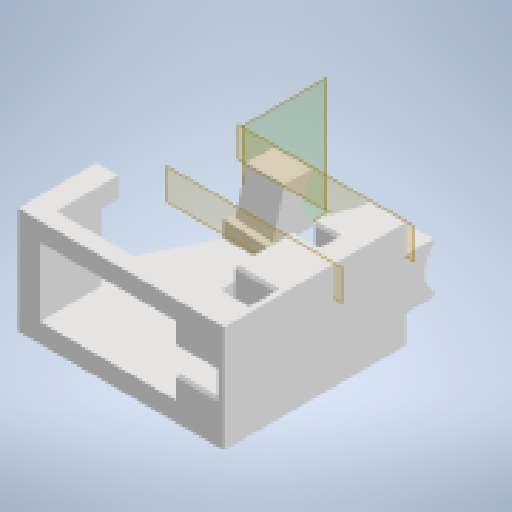
# Autodesk Inventor part: Servo Mount
Saved by Autodesk Inventor 2024 (Build 280153000, 153)
## iProperties
Created: 2024-11-25
Part Number: Servo Mount
Material: Generic
Document SubType Name: Modeling
Designer: Tommy Rohmann
Density: 1 g/cm^3
Appearance: Default
Author: Tommy Rohmann
Autodesk Inventor part; units mm, degrees
sketch "Servo Footprint" plane through (0, 0, 0) normal (0, 0, 1) x (1, 0, 0)
  line L0 (-70.3478, -47.479) -> (-30.4698, -47.479)
  line L1 (-30.4698, -47.479) -> (-30.4698, -27.667)
  line L2 (-30.4698, -27.667) -> (-70.3478, -27.667)
  line L3 (-70.3478, -47.479) -> (-30.4698, -27.667) construction
  line L4 (-30.4698, -47.479) -> (-70.3478, -27.667) construction
  line L5 (-77.5868, -47.479) -> (-23.2308, -47.479)
  line L6 (-23.2308, -47.479) -> (-23.2308, -27.667)
  line L7 (-23.2308, -27.667) -> (-77.5868, -27.667)
  line L8 (-77.5868, -47.479) -> (-23.2308, -27.667) construction
  line L9 (-23.2308, -47.479) -> (-77.5868, -27.667) construction
  line L10 (-30.4698, -37.573) -> (-39.8678, -37.573)
  line L11 (-77.5868, -47.479) -> (-77.5868, -27.667)
  line L12 (-70.3478, -27.667) -> (-70.3478, -47.479)
  point P0 (-45.544, -37.573)
  point P1 (-50.4088, -37.573)
  point P2 (-50.4088, -37.573)
  dimension "d0" = 39.878
  dimension "d1" = 19.812
  dimension "d2" = 54.356
  dimension "d3" = 9.398
  measures "d0" distance of L0.start L0.end
  measures "d1" distance of L1.end L0.end
  measures "d2" distance of L5.start L5.end
  measures "d3" distance of L10.start L10.end
sketch "Valve Casing" plane through (0, 0, 0) normal (0, 0, 1) x (1, 0, 0)
  circle A0 centre (0, 0) radius 8.636
  circle A1 centre (0, 0) radius 11.176
  circle A2 centre (0, 0) radius 12.446
  dimension "d30" = 24.892
  measures "d30" diameter of A2
sketch "Servo Arm Socket" plane through (0, 0, 0) normal (0, 0, 1) x (1, 0, 0)
  arc A0 (4.8166, -0.3016) -> (-4.8166, -0.3016) centre (0, 0) ccw
  line L0 (0, 0) -> (0, -20.32)
  arc A1 (-3.549, -20.5423) -> (3.549, -20.5423) centre (0, -20.32) ccw
  line L1 (-3.549, -20.5423) -> (-4.8166, -0.3016)
  line L2 (4.8166, -0.3016) -> (3.549, -20.5423)
  line L3 (-5.0701, -0.3175) -> (-3.8026, -20.5581)
  arc A2 (-3.8026, -20.5581) -> (3.8026, -20.5581) centre (0, -20.32) ccw
  line L4 (3.8026, -20.5581) -> (5.0701, -0.3175)
  arc A3 (5.0701, -0.3175) -> (-5.0701, -0.3175) centre (0, 0) ccw
  line L5 (-6.3376, -20.7169) -> (-7.6051, -0.4762)
  arc A4 (7.6051, -0.4763) -> (-7.6051, -0.4762) centre (0, 0) ccw
  line L6 (7.6051, -0.4763) -> (6.3376, -20.7169)
  arc A5 (-6.3376, -20.7169) -> (6.3376, -20.7169) centre (0, -20.32) ccw
  dimension "d0" = 39.878
  dimension "d1" = 19.812
  dimension "d2" = 54.356
  dimension "d3" = 9.398
  dimension "d39" = 9.652
  dimension "d40" = 20.32
  dimension "d41" = 7.112
  dimension "d42" = 0.254
  dimension "d43" = 2.54
  measures "d39" diameter of A0
  measures "d40" distance of L0.start L0.end
  measures "d41" diameter of A1
  measures "d42" distance between parallel lines of L1 L3
  measures "d43" distance between parallel lines of L3 L5
sketch "Most Annoying thing Possibly Ever" plane through (0, 0, 0) normal (0, 0, 1) x (1, 0, 0)
  line L0 (1.9811, 57.7148) -> (1.9811, 71.8118)
  line L1 (16.0781, 71.8118) -> (1.9811, 71.8118)
  arc A0 (1.9811, 45.1418) -> (28.6511, 71.8118) centre (1.9811, 71.8118) ccw
  arc A1 (1.9811, 44.6338) -> (29.1591, 71.8118) centre (1.9811, 71.8118) ccw
  circle A2 centre (1.9811, 71.8118) radius 8.636
  circle A3 centre (1.9811, 71.8118) radius 11.176
  circle A4 centre (1.9811, 71.8118) radius 12.446
  arc A5 (6.7977, 71.5101) -> (-2.8354, 71.5101) centre (1.9811, 71.8118) ccw
  line L2 (1.9811, 71.8118) -> (1.9811, 51.4918)
  arc A6 (-1.5679, 51.2695) -> (5.5302, 51.2695) centre (1.9811, 51.4918) ccw
  line L3 (-1.5679, 51.2695) -> (-2.8354, 71.5101)
  line L4 (6.7977, 71.5101) -> (5.5302, 51.2695)
  line L5 (-3.0889, 71.4943) -> (-1.8214, 51.2536)
  arc A7 (-1.8214, 51.2536) -> (5.7837, 51.2536) centre (1.9811, 51.4918) ccw
  line L6 (5.7837, 51.2536) -> (7.0512, 71.4943)
  arc A8 (7.0512, 71.4943) -> (-3.0889, 71.4943) centre (1.9811, 71.8118) ccw
  line L7 (-4.3564, 51.0949) -> (-5.624, 71.3355)
  arc A9 (9.5862, 71.3355) -> (-5.624, 71.3355) centre (1.9811, 71.8118) ccw
  line L8 (9.5862, 71.3355) -> (8.3187, 51.0949)
  arc A10 (-4.3564, 51.0949) -> (8.3187, 51.0949) centre (1.9811, 51.4918) ccw
  arc A11 (2.2828, 76.6283) -> (2.2828, 66.9952) centre (1.9811, 71.8118) ccw
  line L9 (1.9811, 71.8118) -> (22.3011, 71.8118)
  arc A12 (22.5234, 68.2627) -> (22.5234, 75.3608) centre (22.3011, 71.8118) ccw
  line L10 (22.5234, 68.2627) -> (2.2828, 66.9952)
  line L11 (2.2828, 76.6283) -> (22.5234, 75.3608)
  line L12 (2.2986, 66.7417) -> (22.5393, 68.0092)
  arc A13 (22.5393, 68.0092) -> (22.5393, 75.6143) centre (22.3011, 71.8118) ccw
  line L13 (22.5393, 75.6143) -> (2.2986, 76.8818)
  arc A14 (2.2986, 76.8818) -> (2.2986, 66.7417) centre (1.9811, 71.8118) ccw
  line L14 (22.698, 65.4742) -> (2.4574, 64.2067)
  arc A15 (2.4574, 79.4169) -> (2.4574, 64.2067) centre (1.9811, 71.8118) ccw
  line L15 (2.4574, 79.4169) -> (22.698, 78.1493)
  arc A16 (22.698, 65.4742) -> (22.698, 78.1493) centre (22.3011, 71.8118) ccw
  point P0 (7.2472, 66.5457)
  point P1 (1.9811, 48.0247)
  point P2 (25.7682, 71.8118)
  dimension "d61" = 0.508
  measures "d61" radial gap between concentric circles of A0 A1
ref_plane "Work Plane1" through (0, 23.3934, 0) normal (0, 0, 1) x (1, 0, 0)
sketch "Sketch1" plane through (0, 23.3934, 0) normal (0, 0, 1) x (1, 0, 0)
  line L0 (-11.8935, 4.1783) -> (-11.8935, -4.1783) projected
  line L1 (-11.8935, -4.1783) -> (1.6581, -4.1783) projected
  arc A0 (22.129, -4.1783) -> (1.6581, -4.1783) centre (11.8935, -11.6967) ccw projected
  line L2 (35.6806, -4.1783) -> (22.129, -4.1783) projected
  line L3 (35.6806, 4.1783) -> (35.6806, -4.1783) projected
  line L4 (-11.8935, 4.1783) -> (35.6806, 4.1783) projected
  arc A1 (1.6581, -19.2151) -> (22.129, -19.2151) centre (11.8935, -11.6967) ccw projected
  line L5 (1.6581, -19.2151) -> (-11.8935, -19.2151) projected
  line L6 (-11.8935, -19.2151) -> (-11.8936, -27.5717) projected
  line L7 (-11.8936, -27.5717) -> (35.6806, -27.5717) projected
  line L8 (35.6806, -19.2151) -> (35.6806, -27.5717) projected
  line L9 (22.129, -19.2151) -> (35.6806, -19.2151) projected
  line L10 (35.6806, -19.2151) -> (35.6806, -4.1783) projected
  line L11 (-11.8935, -19.2151) -> (-11.8935, -4.1783) projected
  arc A2 (1.278, -18.668) -> (18.8649, -1.0811) centre (11.8935, -11.6967) ccw
  circle A3 centre (11.8936, -11.6967) radius 27.178
  line L12 (18.8649, -1.0811) -> (18.8649, 14.572)
  line L13 (1.278, -18.668) -> (-14.3751, -18.668)
  circle A4 centre (11.8936, -11.6967) radius 12.7
  line L14 (-11.8935, -19.2151) -> (-11.8935, -17.0166)
  line L15 (0.3239, -16.5227) -> (0.3239, -19.2151)
  line L16 (-11.8935, -19.2151) -> (0.3239, -19.2151)
  circle A5 centre (-8.4264, -11.6967) radius 6.35
  line L17 (-8.8233, -18.0343) -> (0.3239, -18.6071)
  point P0 (0, -23.3934)
  point P1 (18.8649, 4.1783)
  point P2 (22.129, -4.1783)
  point P3 (18.8649, -1.0811)
  constraints: 13 end point, 4 point on circle, 3 centre point, 2 coincident, 2 vertical, 1 collinear, 1 concentric, 1 parallel, 1 perpendicular, 1 point on line, 5 other
ref_plane "Work Plane2" through (0, 23.3934, 21.463) normal (0, 0, 1) x (1, 0, 0)
sketch "Sketch2" plane through (0, 23.3934, 21.463) normal (0, 0, 1) x (1, 0, 0)
  line L0 (-18.5864, -1.7907) -> (-18.5864, -21.6027)
  line L1 (-25.8254, -1.7907) -> (-25.8254, -21.6027)
  line L2 (35.6806, -27.5717) -> (-25.8255, -27.5717)
  line L3 (-25.8255, -27.5717) -> (-25.8255, 4.1783)
  line L4 (-25.8255, 4.1783) -> (35.6806, 4.1783)
  line L5 (35.6806, -27.5717) -> (35.6806, 4.1783)
  line L6 (21.2916, -1.7907) -> (21.2916, 4.1783)
  line L7 (-18.5864, -1.7907) -> (-18.5864, 4.1783)
  line L8 (28.5305, -1.7907) -> (28.5305, 4.1783)
  line L9 (-18.5864, -21.6027) -> (21.2916, -21.6027)
  line L10 (21.2916, -21.6027) -> (21.2916, -1.7907)
  line L11 (21.2916, -1.7907) -> (-18.5864, -1.7907)
  line L12 (-18.5864, -21.6027) -> (21.2916, -1.7907) construction
  line L13 (21.2916, -21.6027) -> (-18.5864, -1.7907) construction
  line L14 (-25.8254, -21.6027) -> (28.5306, -21.6027)
  line L15 (28.5306, -21.6027) -> (28.5306, -1.7907)
  line L16 (28.5306, -1.7907) -> (-25.8254, -1.7907)
  line L17 (-25.8254, -21.6027) -> (28.5306, -1.7907) construction
  line L18 (28.5306, -21.6027) -> (-25.8254, -1.7907) construction
  line L19 (21.2916, -11.6967) -> (11.8936, -11.6967)
  line L20 (-25.8254, -21.6027) -> (-25.8254, -1.7907)
  line L21 (-18.5864, -1.7907) -> (-18.5864, -21.6027)
  point P0 (0, -23.3934)
  point P1 (11.8935, -11.6967)
  point P2 (-25.8254, -1.7907)
  point P3 (-25.8254, -1.7907)
  point P4 (21.2916, -21.6027)
  point P5 (-25.8254, -1.7907)
  point P6 (21.2916, -21.6027)
  constraints: 18 end point, 4 vertical, 3 perpendicular, 3 point on line, 1 horizontal, 8 other
ref_plane "Work Plane5" through (-11.8935, 19.2151, 0) normal (0, 0, 1) x (1, 0, 0)
ref_plane "Work Plane6" through (0.3782, 20.624, 2.413) normal (0, 0, -1) x (-0.1736598, 0.9848057, 0)
ref_plane "Work Plane7" through (-11.8935, 11.6967, -13.335) normal (-1, 0, 0) x (0, -1, 0)
sketch "Sketch7" plane through (-11.8935, 11.6967, -13.335) normal (-1, 0, 0) x (0, -1, 0)
  line L0 (-15.875, -9.525) -> (15.875, -9.525) projected
  line L1 (15.875, -9.525) -> (15.875, 13.335) projected
  line L2 (7.5184, 13.335) -> (15.875, 13.335) projected
  line L3 (7.5184, -1.1176) -> (7.5184, 13.335) projected
  arc A0 (-7.5184, -1.1176) -> (7.5184, -1.1176) centre (0, -1.1176) ccw projected
  line L4 (-7.5184, -1.1176) -> (-7.5184, 13.335) projected
  line L5 (-15.875, 13.335) -> (-7.5184, 13.335) projected
  line L6 (-15.875, -9.525) -> (-15.875, 13.335) projected
  line L7 (0, -1.1176) -> (0, 0.1524)
  arc A1 (5.9368, 4.9293) -> (-5.9368, 4.9293) centre (0, 0.1524) ccw
  line L8 (7.5184, 5.4866) -> (7.5184, 13.335)
  line L9 (-7.5184, 5.4866) -> (-7.5184, 13.335)
  arc A2 (5.9368, 4.9293) -> (7.5184, 5.4866) centre (6.6294, 5.4866) ccw
  arc A3 (-7.5184, 5.4866) -> (-5.9368, 4.9293) centre (-6.6294, 5.4866) ccw
  line L10 (0, 8.7376) -> (15.875, 8.7376)
  line L11 (0, 12.065) -> (15.875, 12.065)
  line L12 (-9.9274, 15.748) -> (-19.4435, 15.748) projected
  line L13 (-15.875, 15.748) -> (15.875, 15.748) construction
  line L14 (15.875, 15.748) -> (15.875, 13.335)
  line L15 (7.5184, 13.335) -> (15.875, 13.335)
  line L16 (-15.875, 15.748) -> (-15.875, 13.335)
  line L17 (-7.5184, 13.335) -> (-15.875, 13.335)
  line L18 (-15.875, 15.24) -> (15.875, 15.24)
  line L19 (0, 15.24) -> (-7.5184, 13.335)
  line L20 (-15.875, 13.335) -> (-7.5184, 13.335)
  line L21 (0, 15.24) -> (-7.5184, 13.335)
  line L22 (-15.875, 15.24) -> (0, 15.24)
  line L23 (-15.875, 13.335) -> (-15.875, 15.24)
  point P0 (11.6967, 13.335)
  point P1 (-7.5184, 1.3926)
  point P2 (7.5184, 1.3926)
  point P3 (-7.5184, 5.4866)
  dimension "d51" = 1.27
  dimension "d52" = 15.24
  dimension "d53" = 0.889
  dimension "d54" = 3.3274
  dimension "d55" = 0.508
  dimension "d56" = 1.27
  constraints: 32 end point, 8 point on circle, 8 point on line, 7 collinear, 5 perpendicular, 4 tangent, 3 centre point, 1 coincident, 1 equal radius, 1 horizontal, 1 midpoint, 1 parallel, 1 vertical
  measures "d51" distance of L7.start L7.end
  measures "d52" diameter of A1
  measures "d53" radius of A2
  measures "d54" distance between parallel lines of L10 L11
  measures "d55" distance between parallel lines of L13 L18
  measures "d56" distance between parallel lines of L2 L11
ref_plane "Work Plane8" through (35.6806, -4.1783, -22.86) normal (1, 0, 0) x (0, 1, 0)
extrude "Extrusion10" add sketch "Sketch7" against normal up to surface (47.5742 mm away) contours L16 L18 L19 L5 | L19 L18 L14 L2 L3 A2 A1 A3 L4
ref_plane "Work Plane9" through (-11.8935, 19.2151, 0) normal (0, 0, 1) x (1, 0, 0)
extrude "Extrusion14" add sketch "Sketch2" along normal blind 20.574 contours L16 L3 L4 L7 | L0 L14 L1 L16 | L9 L14 L15 L8 L4 L5 L2 L3 | L16 L15 L14 L10 | L6 L4 L8 L16
extrude "Extrusion15" cut sketch "Sketch2" along normal blind 14.224 contours L7 L4 L6 L11 | L0 L14 L1 L16 | L16 L15 L14 L10
extrude "Extrusion16" cut sketch "Sketch2" along normal blind 9.144 contours L16 L3 L4 L7 | L6 L4 L8 L16
extrude "Extrusion17" add sketch "Sketch2" along normal blind 4.064 contours L6 L4 L8 L16
extrude "Extrusion18" add sketch "Sketch2" against normal up to surface (19.558 mm away) contours L9 L14 L15 L8 L4 L5 L2 L3 | L6 L4 L8 L16
sketch "Sketch10" plane through (-11.8935, 27.5717, 0) normal (0, 1, 0) x (1, 0, 0)
  line L0 (36.2331, -21.463) -> (36.2331, 3.81)
  line L1 (11.3411, -21.463) -> (11.3411, 3.81)
  line L2 (11.3411, -21.463) -> (11.3411, 12.3467)
  line L3 (11.3411, 12.3467) -> (36.2331, 12.3467)
  line L4 (36.2331, 12.3467) -> (36.2331, -21.463)
  line L5 (36.2331, -21.463) -> (36.2331, -22.733)
  line L6 (36.2331, -22.733) -> (11.3411, -22.733)
  line L7 (11.3411, -22.733) -> (11.3411, -21.463)
  line L8 (36.2331, -22.733) -> (36.7411, -22.733)
  line L9 (36.7411, -22.733) -> (36.7411, 12.3467)
  line L10 (36.7411, 12.3467) -> (36.2331, 12.3467)
  point P0 (11.8935, 0)
  point P1 (11.3411, 3.81)
  point P2 (36.2331, 3.81)
  dimension "d84" = 1.27
  dimension "d87" = 0.508
  constraints: 22 end point, 5 perpendicular, 3 point on line, 2 vertical, 1 collinear, 1 horizontal, 4 other
  measures "d84" distance of L0.start L5.end
  measures "d87" distance of L5.end L8.end
extrude "Extrusion22" cut sketch "Sketch10" against normal up to surface (25.781 mm away)
extrude "Extrusion23" cut sketch "Sketch1" along normal blind 25.4 contours A0 A2 A1 A4
sketch "Sketch11" plane through (-11.8935, 11.6967, -13.335) normal (-1, 0, 0) x (0, 0, 1)
  line L0 (13.335, 15.875) -> (13.335, 7.3279)
  line L1 (13.335, 7.3279) -> (15.24, 0)
  line L2 (15.24, 2.5273) -> (15.24, -2.5273) projected
  line L3 (15.24, 2.5273) -> (15.24, 15.875) projected
  line L4 (15.24, 0) -> (15.24, 15.875)
  line L5 (15.24, 15.875) -> (13.335, 15.875)
  line L6 (13.335, 6.609) -> (15.24, -0.7188)
  line L7 (15.24, 0) -> (15.24, -0.7188)
  line L8 (13.335, 6.609) -> (13.335, 8.747)
  point P0 (13.335, -11.6967)
  point P1 (13.335, 7.3279)
  constraints: 14 end point, 2 point on line, 2 vertical, 1 collinear, 1 midpoint, 1 perpendicular
extrude "Extrusion24" cut sketch "Sketch11" against normal blind 25.4
sketch "Sketch12" plane through (-11.8935, -4.1783, 0) normal (0, -1, 0) x (1, 0, 0)
  line L0 (-13.9319, 30.607) -> (-6.6929, 30.607) projected
  line L1 (0, 1.905) -> (11.3411, 1.905) projected
  line L2 (0, 1.905) -> (-13.9319, 30.607)
  line L3 (-13.9319, 35.687) -> (-13.9319, 1.905) projected
  line L4 (-13.9319, 1.905) -> (-13.9319, 30.607)
  line L5 (0, 1.905) -> (-13.9319, 1.905)
  point P0 (11.8935, 0)
  constraints: 6 end point, 1 collinear, 1 perpendicular
extrude "Extrusion25" cut sketch "Sketch12" against normal blind 36.5125
sketch "Sketch13" plane through (-11.8935, -4.1783, 0) normal (0, -1, 0) x (1, 0, 0)
  line L0 (15.8397, 25.4) -> (15.8397, 0) projected
  line L1 (31.7345, 0) -> (31.7345, 25.4) projected
  line L2 (0, 0) -> (47.5742, 0) projected
  line L3 (11.3411, -7.8484) -> (11.3411, 0) projected
  line L4 (36.7411, 0) -> (36.7411, -7.8484) projected
  line L5 (11.3411, 0) -> (11.3411, 25.4)
  line L6 (11.3411, 25.4) -> (36.7411, 25.4)
  line L7 (36.7411, 0) -> (36.7411, 22.733) projected
  line L8 (36.7411, 25.4) -> (36.7411, 0)
  line L9 (36.7411, 0) -> (11.3411, 0)
  point P0 (11.8935, 0)
  constraints: 8 end point, 2 perpendicular, 1 collinear, 1 point on line
extrude "Extrusion26" cut sketch "Sketch13" against normal blind 23.8125
fillet "Fillet1" radius 3.175 2 edges at (24.8475, -1.1938, 25.4) (-0.5524, -1.1938, 25.4)
sketch "Sketch14" plane through (21.2916, 27.5717, 42.037) normal (0, 1, 0) x (1, 0, 0)
  line L0 (7.239, 16.51) -> (7.239, 40.132) projected
  line L1 (3.556, 42.037) -> (3.556, 19.304) projected
  line L2 (3.556, 19.304) -> (0, 19.304) projected
  line L3 (0, 19.304) -> (0, 16.51) projected
  line L4 (7.239, 16.51) -> (0, 16.51) projected
  line L5 (7.239, 16.51) -> (7.239, 11.43) projected
  line L6 (7.239, 11.43) -> (0, 11.43) projected
  line L7 (0, 11.43) -> (0, 0) projected
  line L8 (14.3891, 0) -> (0, 0) projected
  line L9 (14.3891, 42.037) -> (14.3891, 0) projected
  line L10 (3.556, 42.037) -> (14.3891, 42.037) projected
  line L11 (0, 11.43) -> (0, 16.51)
  line L12 (0, 16.51) -> (0, 23.368)
  line L13 (0, 23.368) -> (7.239, 23.368)
  line L14 (7.239, 16.51) -> (7.239, 11.43)
  line L15 (0, 16.51) -> (7.239, 16.51)
  line L16 (7.239, 23.368) -> (7.239, 28.448)
  line L17 (7.239, 28.448) -> (0, 28.448)
  line L18 (3.556, 40.132) -> (7.239, 40.132) projected
  line L19 (0, 28.448) -> (3.556, 40.132)
  point P0 (-21.2916, 42.037)
  point P1 (3.556, 23.368)
  point P2 (3.556, 28.448)
  dimension "d97" = 6.858
  dimension "d98" = 5.08
  constraints: 16 end point, 4 perpendicular, 4 point on line, 1 collinear
  measures "d97" distance of L3.end L12.end
  measures "d98" distance of L13.end L16.end
extrude "Extrusion27" cut sketch "Sketch14" against normal up to surface (5.969 mm away) contours L4 L3 L2 L1 L13 L0 | L0 L18 L1 L10 L9 L8 L7 L6 L5 | L13 L1 L17 L0 | L17 L1 L18 L0 | L1 L2 L12 L13
extrude "Extrusion28" add sketch "Sketch14" against normal up to surface (5.969 mm away) contours L4 L3 L2 L1 L13 L0 | L5 L6 L11 L4 | L0 L18 L1 L10 L9 L8 L7 L6 L5 | L17 L1 L18 L0 | L1 L2 L12 L13 | L17 L19 L1
extrude "Extrusion29" add sketch "Sketch14" against normal up to surface (25.781 mm away) contours L17 L1 L18 L0
sketch "Sketch15" plane through (-18.5864, 1.7907, 42.037) normal (1, 0, 0) x (0, 0, -1)
  line L0 (11.43, 19.812) -> (11.43, 25.781) projected
  line L1 (11.43, 25.781) -> (0, 25.781) projected
  line L2 (0, 0) -> (0, 25.781) projected
  line L3 (6.35, 0) -> (0, 0) projected
  line L4 (6.35, 0) -> (6.35, 19.812) projected
  line L5 (11.43, 19.812) -> (6.35, 19.812) projected
  point P0 (42.037, -1.7907)
extrude "Extrusion30" cut sketch "Sketch15" against normal blind 0.508
sketch "Sketch16" plane through (0, 23.3934, 42.037) normal (0, 0, 1) x (1, 0, 0)
  line L0 (-19.0945, -21.6027) -> (-19.0945, 4.1783) projected
  line L1 (-19.0945, 4.1783) -> (-25.8255, 4.1783) projected
  line L2 (-25.8255, 4.1783) -> (-25.8255, -27.5717) projected
  line L3 (-25.8255, -27.5717) -> (35.6806, -27.5717) projected
  line L4 (35.6806, -27.5717) -> (35.6806, 4.1783) projected
  line L5 (21.2916, 4.1783) -> (35.6806, 4.1783) projected
  line L6 (21.2916, 4.1783) -> (21.2915, -21.6027) projected
  line L7 (21.2915, -21.6027) -> (-19.0945, -21.6027) projected
  line L8 (35.6806, -11.6967) -> (-25.8255, -11.6967)
  line L9 (21.2915, -15.1892) -> (35.6806, -15.1892)
  line L10 (21.2916, -8.2042) -> (35.6806, -8.2042)
  line L11 (28.1495, -15.1892) -> (28.1495, 4.1783)
  line L12 (-19.0945, -1.7907) -> (-25.8254, -1.7907) projected
  line L13 (-25.8254, -1.7907) -> (-19.0945, -1.7907) projected
  line L14 (28.5305, -1.7907) -> (21.2916, -1.7907) projected
  line L15 (28.5305, -1.7907) -> (21.2916, -1.7907) projected
  line L16 (-25.8254, -1.7907) -> (35.6806, -1.7907)
  line L17 (35.6806, 4.1783) -> (-25.8255, 4.1783)
  point P0 (0, -23.3934)
  point P1 (28.1495, -8.2042)
  dimension "d110" = 6.985
  dimension "d111" = 3.4925
  constraints: 12 end point, 7 point on line, 4 perpendicular, 2 midpoint, 1 horizontal
  measures "d110" distance between parallel lines of L10 L9
  measures "d111" distance between parallel lines of L8 L9
extrude "Extrusion31" add sketch "Sketch16" along normal blind 12.065 contours L12 L2 L1 L0 | L0 L8 L2 L12 | L0 L17 L6 L16 | L0 L7 L6 L9 L4 L3 L2 L8 | L14 L11 L10 L6 | L6 L5 L11 L14 | L8 L11 L9 L6 | L6 L10 L11 L8 | L14 L16 L4 L10 L11 | L11 L5 L4 L16 L14 | L11 L10 L4 L8 | L8 L4 L9 L11
extrude "Extrusion32" cut sketch "Sketch16" along normal blind 7.112 contours L0 L17 L6 L16
extrude "Extrusion33" cut sketch "Sketch16" along normal blind 4.699 contours L14 L11 L10 L6 | L6 L5 L11 L14 | L8 L11 L9 L6 | L6 L10 L11 L8
extrude "Extrusion34" cut sketch "Sketch16" along normal blind 20.574 contours L8 L11 L9 L6 | L6 L10 L11 L8
sketch "Sketch17" plane through (-0.5524, 1.7907, 1.905) normal (0, 0, 1) x (1, 0, 0)
  line L0 (-8.2709, 3.5684) -> (0.8763, 2.9956) projected
  circle A0 centre (-7.874, 9.906) radius 6.35 projected
  line L1 (0, 0) -> (0, 7.3787) projected
  line L2 (21.844, 0) -> (-18.542, 0) projected
  line L3 (-11.3411, 0) -> (-11.3411, 9.1872) projected
  line L4 (0, 3.0505) -> (-11.3411, 3.7607)
  line L5 (0, 2.796) -> (-11.357, 3.5072)
  line L6 (-11.3411, 3.5062) -> (-11.3411, 0)
  line L7 (-11.3411, 0) -> (0, 0)
  line L8 (0, 2.796) -> (0, 0)
  line L9 (-11.3411, 3.7607) -> (0, 3.0505)
  line L10 (-11.3411, 4.7787) -> (0, 4.0685)
  line L11 (0, 4.0685) -> (0, 2.796)
  line L12 (-11.3411, 4.7787) -> (-11.3411, 3.5062)
  point P0 (0.5524, -1.7907)
  point P1 (-11.3411, 9.906)
  point P2 (0, 2.796)
  dimension "d124" = 0.254
  dimension "d133" = 1.27
  constraints: 18 end point, 8 point on line, 4 collinear, 3 parallel, 1 perpendicular, 1 other
  measures "d124" distance between parallel lines of L4 L5
  measures "d133" distance between parallel lines of L10 L5
extrude "Extrusion35" add sketch "Sketch17" along normal up to surface (11.684 mm away) contours A0 L10 L1 L0 | L4 L3 A0 | A0 L3 L10 | L0 L1 L5 L3 L4 | L1 L2 L3 L5 picked at (-7.3291, 4.3413)
sketch "Sketch18" plane through (21.2916, 1.7907, 35.687) normal (0, 1, 0) x (1, 0, 0)
  line L0 (-33.1851, 22.098) -> (-33.1851, 33.782) projected
  line L1 (-33.1851, 33.782) -> (-47.117, 5.08) projected
  line L2 (-47.117, 0) -> (-47.117, 5.08) projected
  line L3 (-47.117, 0) -> (-40.386, 0) projected
  line L4 (-40.386, 0) -> (-40.386, -18.415) projected
  line L5 (0, -18.415) -> (-40.386, -18.415) projected
  line L6 (0, 0) -> (0, -18.415) projected
  line L7 (0, 0) -> (7.239, 0) projected
  line L8 (7.239, 22.098) -> (7.239, 0) projected
  line L9 (7.239, 22.098) -> (3.556, 22.098) projected
  line L10 (3.556, 22.098) -> (3.556, 13.462) projected
  arc A0 (0.381, 10.287) -> (3.556, 13.462) centre (0.381, 13.462) ccw projected
  line L11 (0.381, 10.287) -> (-18.669, 10.287) projected
  arc A1 (-21.844, 13.462) -> (-18.669, 10.287) centre (-18.669, 13.462) ccw projected
  line L12 (-21.844, 13.462) -> (-21.844, 22.098) projected
  line L13 (-21.844, 22.098) -> (-33.1851, 22.098) projected
  line L14 (-33.1851, 22.098) -> (-38.8565, 22.098)
  line L15 (-38.8565, 22.098) -> (-33.1851, 33.782)
  line L16 (-33.1851, 33.782) -> (-33.1851, 22.098)
  point P0 (-21.2916, 35.687)
  constraints: 6 end point, 1 collinear, 1 horizontal, 1 point on line
extrude "Extrusion36" add sketch "Sketch18" along normal up to surface (4.7787 mm away) contours L14 L1 L0
sketch "Sketch19" plane through (-11.8935, 11.6967, -13.335) normal (-1, 0, 0) x (0, 0, 1)
  line L0 (15.24, -15.875) -> (15.24, -5.1273) projected
  line L1 (15.24, -5.1273) -> (15.24, -0.7188) projected
  line L2 (13.335, 6.609) -> (13.335, 7.5184) projected
  line L3 (13.335, 7.5184) -> (5.4866, 7.5184) projected
  arc A0 (5.4866, 7.5184) -> (4.9293, 5.9368) centre (5.4866, 6.6294) ccw projected
  arc A1 (4.9293, -5.9368) -> (4.9293, 5.9368) centre (0.1524, 0) ccw projected
  arc A2 (4.9293, -5.9368) -> (5.4866, -7.5184) centre (5.4866, -6.6294) ccw projected
  line L4 (5.4866, -7.5184) -> (13.335, -7.5184) projected
  line L5 (13.335, -7.5184) -> (13.335, -15.875) projected
  line L6 (13.335, -15.875) -> (15.24, -15.875) projected
  line L7 (15.24, -15.875) -> (15.24, -5.1273) projected
  line L8 (43.942, -15.875) -> (15.24, -15.875) projected
  line L9 (43.942, -9.906) -> (43.942, -15.875) projected
  line L10 (26.924, -9.906) -> (43.942, -9.906) projected
  line L11 (26.924, -9.906) -> (26.924, -5.1273) projected
  line L12 (26.924, -5.1273) -> (15.24, -5.1273) projected
  line L13 (15.24, -5.1273) -> (16.51, -5.1273)
  line L14 (16.51, -5.1273) -> (13.335, 7.5184)
  line L15 (16.51, -5.1273) -> (15.24, -5.1273)
  line L16 (15.24, -5.1273) -> (15.24, -15.875)
  line L17 (15.24, -15.875) -> (13.335, -15.875)
  line L18 (13.335, -15.875) -> (13.335, 7.5184)
  line L19 (16.51, -5.1273) -> (16.51, -15.875)
  line L20 (43.942, -15.875) -> (15.24, -15.875) projected
  line L21 (16.51, -15.875) -> (15.24, -15.875)
  line L22 (13.335, 7.5184) -> (19.9572, 7.5184)
  line L23 (19.9572, 7.5184) -> (16.51, -5.1273)
  line L24 (15.24, -0.7188) -> (13.335, 6.609) projected
  point P0 (13.335, -11.6967)
  dimension "d134" = 1.27
  constraints: 20 end point, 3 collinear, 2 horizontal, 2 perpendicular, 2 point on line
  measures "d134" distance of L7.end L13.end
extrude "Extrusion37" add sketch "Sketch19" against normal up to surface (11.3411 mm away) contours L6 L5 L18 L24 L1 L0 | L0 L12 L19 L8 | L1 L24 L2 L14 L12
sketch "Sketch21" plane through (28.1496, 8.2042, 42.037) normal (-1, 0, 0) x (0, 0, 1)
  line L0 (4.699, 6.985) -> (4.699, 19.3675) projected
  line L1 (0, 19.3675) -> (4.699, 19.3675) projected
  line L2 (0, 0) -> (0, 19.3675) projected
  line L3 (0, 0) -> (12.065, 0) projected
  line L4 (12.065, 6.985) -> (12.065, 0) projected
  line L5 (4.699, 6.985) -> (12.065, 6.985) projected
  line L6 (-28.448, 19.3675) -> (-28.448, -6.4135) projected
  line L7 (-28.448, -6.4135) -> (-6.35, -6.4135) projected
  line L8 (-6.35, -6.4135) -> (-6.35, 13.3985) projected
  line L9 (-6.35, 13.3985) -> (-23.368, 13.3985) projected
  line L10 (-23.368, 19.3675) -> (-23.368, 13.3985) projected
  line L11 (-28.448, 19.3675) -> (-23.368, 19.3675) projected
  point P0 (-42.037, -8.2042)
extrude "Extrusion38" cut sketch "Sketch21" against normal blind 0.508
sketch "Sketch22" plane through (0, 23.3934, 42.037) normal (0, 0, 1) x (1, 0, 0)
  line L0 (21.2916, 4.1783) -> (28.6576, 4.1783) projected
  line L1 (21.2915, -15.1892) -> (21.2916, 4.1783) projected
  line L2 (21.2915, -15.1892) -> (28.6576, -15.1892) projected
  line L3 (28.6576, -15.1892) -> (28.6576, 4.1783) projected
  point P0 (0, -23.3934)
extrude "Extrusion39" cut sketch "Sketch21" against normal blind 5.08 contours L5 L4 L3 L2 L1 L0
extrude "Extrusion40" cut sketch "Sketch22" against normal blind 5.334
sketch "Sketch23" plane through (-17.5649, 1.7907, 13.589) normal (0, 0, 1) x (1, 0, 0)
  line L0 (5.6714, 4.7787) -> (17.0125, 4.0685) projected
  line L1 (5.6714, 4.7787) -> (0, 4.7787) projected
  line L2 (0, 0) -> (0, 4.7787) projected
  line L3 (17.0125, 0) -> (0, 0) projected
  line L4 (17.0125, 4.0685) -> (17.0125, 0) projected
  point P0 (17.5649, -1.7907)
extrude "Extrusion41" cut sketch "Sketch23" against normal blind 8.3312
extrude "Extrusion42" cut sketch "Sketch21" against normal up to surface (0.508 mm away) contours L5 L4 L3 L2 L1 L0
sketch "Sketch24" plane through (0, 23.3934, 42.037) normal (0, 0, 1) x (1, 0, 0)
  line L0 (28.6576, 4.1783) -> (28.6576, -15.1892) projected
  line L1 (28.6576, -15.1892) -> (33.2295, -15.1892) projected
  line L2 (33.2295, -15.1892) -> (33.2295, 4.1783) projected
  line L3 (28.6576, 4.1783) -> (33.2295, 4.1783) projected
  point P0 (0, -23.3934)
extrude "Extrusion43" cut sketch "Sketch24" against normal up to surface (5.334 mm away)
sketch "Sketch25" plane through (0, 23.3934, 46.736) normal (0, 0, -1) x (-1, 0, 0)
  line L0 (-33.2295, -8.2042) -> (-21.2916, -8.2042) projected
  line L1 (-21.2916, 4.1783) -> (-21.2916, -8.2042) projected
  line L2 (-33.2295, 4.1783) -> (-21.2916, 4.1783) projected
  line L3 (-33.2295, 4.1783) -> (-33.2295, -8.2042) projected
  point P0 (0, -23.3934)
extrude "Extrusion44" add sketch "Sketch25" along normal blind 2.54
sketch "Sketch26" plane through (-25.8254, 1.7907, 35.687) normal (0, 1, 0) x (1, 0, 0)
  line L0 (54.483, 22.098) -> (50.673, 22.098) projected
  line L1 (50.673, 22.098) -> (50.673, 13.462) projected
  arc A0 (47.498, 10.287) -> (50.673, 13.462) centre (47.498, 13.462) ccw projected
  line L2 (47.498, 10.287) -> (28.448, 10.287) projected
  arc A1 (25.273, 13.462) -> (28.448, 10.287) centre (28.448, 13.462) ccw projected
  line L3 (25.273, 13.462) -> (25.273, 30.4292) projected
  line L4 (25.273, 30.4292) -> (12.3045, 30.4292) projected
  line L5 (12.3045, 30.4292) -> (0, 5.08) projected
  line L6 (0, 0) -> (0, 5.08) projected
  line L7 (0, 0) -> (6.731, 0) projected
  line L8 (6.731, 0) -> (6.731, -18.415) projected
  line L9 (47.117, -18.415) -> (6.731, -18.415) projected
  line L10 (47.117, 0) -> (47.117, -18.415) projected
  line L11 (47.117, 0) -> (54.483, 0) projected
  line L12 (54.483, 0) -> (54.483, 22.098) projected
  point P0 (25.8255, 35.687)
extrude "Extrusion45" cut sketch "Sketch26" against normal blind 0.254
sketch "Sketch27" plane through (21.2916, 21.6027, 18.669) normal (-1, 0, 0) x (0, 0, 1)
  line L0 (17.018, -20.066) -> (35.433, -20.066) projected
  line L1 (35.433, -13.3985) -> (35.433, -20.066) projected
  line L2 (35.433, -13.3985) -> (18.034, -13.3985) projected
  line L3 (18.034, -13.3985) -> (18.034, 5.969) projected
  line L4 (0, 5.969) -> (18.034, 5.969) projected
  line L5 (0, 5.969) -> (0, 0) projected
  line L6 (0, 0) -> (17.018, 0) projected
  line L7 (17.018, 0) -> (17.018, -20.066) projected
  line L8 (25.527, -6.4135) -> (35.433, -6.4135) projected
  line L9 (35.433, 0) -> (35.433, -6.4135) projected
  line L10 (30.48, 0) -> (35.433, 0) projected
  line L11 (30.48, 0) -> (30.48, 5.969) projected
  line L12 (25.527, 5.969) -> (30.48, 5.969) projected
  line L13 (25.527, -6.4135) -> (25.527, 5.969) projected
  point P0 (-18.669, -21.6027)
extrude "Extrusion46" cut sketch "Sketch27" against normal blind 0.254
sketch "Sketch28" plane through (-19.0944, 21.6027, 49.149) normal (0, -1, 0) x (1, 0, 0)
  line L0 (0, 0) -> (40.64, 0) projected
  line L1 (40.64, 0) -> (40.64, 4.953) projected
  line L2 (0, 4.953) -> (40.64, 4.953) projected
  line L3 (0, 0) -> (0, 4.953) projected
  point P0 (19.0944, -49.149)
extrude "Extrusion47" cut sketch "Sketch28" against normal blind 0.508
sketch "Sketch29" plane through (-19.0944, 1.7907, 42.037) normal (1, 0, 0) x (0, 0, -1)
  line L0 (11.43, 19.812) -> (6.35, 19.812) projected
  line L1 (11.43, 25.781) -> (11.43, 19.812) projected
  line L2 (-7.112, 25.781) -> (11.43, 25.781) projected
  line L3 (-7.112, 25.781) -> (-7.112, 20.32) projected
  line L4 (-7.112, 20.32) -> (-12.065, 20.32) projected
  line L5 (-12.065, -0.254) -> (-12.065, 20.32) projected
  line L6 (-12.065, -0.254) -> (6.35, -0.254) projected
  line L7 (6.35, 19.812) -> (6.35, -0.254) projected
  point P0 (42.037, -1.7907)
extrude "Extrusion48" cut sketch "Sketch29" against normal blind 0.254
chamfer "Chamfer4" distance 0.762 angle 45 10 edges at (27.3876, 27.5717, 36.703) (33.2296, 27.5717, 40.4495) (27.3876, 27.5717, 44.196) (25.1016, 27.5717, 18.669) (28.6576, 27.5717, 16.129) (24.9746, 27.5717, 13.589) (21.2916, 24.5872, 13.589) (33.2296, 11.6967, 54.102) (27.3875, 8.2042, 54.102) (27.3876, 15.1892, 54.102)
equation "\"d111\" = 0.5 * d110"
body "Solid3"
